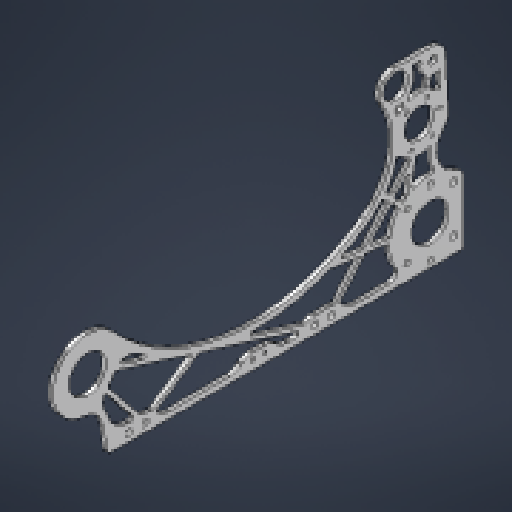
# Autodesk Inventor part: PLATE,SHOOTER,SIDE
Saved by Autodesk Inventor 2026 (Build 300175000, 175)
## iProperties
Created: 2026-01-27
Part Number: PLATE,SHOOTER,SIDE
Material: Aluminum 6061
Document SubType Name: Sheet Metal
Designer: Owen L
Density: 2.7 g/cm^3
Sheet Metal Rule: Default
Appearance: Aluminum - Flat
Mass: 86.5939 g
Surface Area: 289.582 cm^2
Volume: 32.0718 cm^3
Author: Owen L
Autodesk Inventor part; units mm, degrees
ref_plane "YZ Plane" through (0, 0, 0) normal (1, 0, 0) x (0, 1, 0)
ref_plane "XZ Plane" through (0, 0, 0) normal (0, 1, 0) x (-1, 0, 0)
ref_plane "XY Plane" through (0, 0, 0) normal (0, 0, 1) x (1, 0, 0)
sketch "Sketch1" plane through (0, 0, 0) normal (1, 0, 0) x (0, 0, -1)
  circle A0 centre (0, 0) radius 50.8 construction
  arc A1 (166.896579, -77.825153) -> (181.352348, 31.977312) centre (0, 0) ccw construction
  line L0 (0, 0) -> (181.352348, 31.977312) construction
  line L1 (0, 0) -> (184.15, 0) construction
  line L2 (0, 0) -> (166.896579, -77.825153) construction
  arc A2 (207.917963, -26.102167) -> (206.366465, 36.387976) centre (0, 0) ccw construction
  line L3 (0, 0) -> (207.917963, -26.102167) construction
  line L4 (0, 0) -> (206.366465, 36.387976) construction
  circle A3 centre (206.366465, 36.387976) radius 25.4 construction
  circle A4 centre (207.917963, -26.102167) radius 25.4 construction
  arc A5 (206.366465, 36.387976) -> (148.174226, 148.174226) centre (0, 0) ccw construction
  line L5 (0, 0) -> (148.174226, 148.174226) construction
  line L6 (0, 0) -> (206.366465, 36.387976) construction
  arc A6 (185.021668, 98.377766) -> (148.174226, 148.174226) centre (0, 0) ccw construction
  line L7 (0, 0) -> (185.021668, 98.377766) construction
  line L8 (0, 0) -> (148.174226, 148.174226) construction
  circle A7 centre (185.021668, 98.377766) radius 25.4 construction
  circle A8 centre (148.174226, 148.174226) radius 25.4 construction
  circle A9 centre (236.638695, 73.025) radius 15.24 construction
  line L9 (238.323441, -60.809535) -> (238.323441, -0.484535) construction
  line L10 (238.323441, -0.484535) -> (289.123441, -0.484535) construction
  line L11 (289.123441, -0.484535) -> (289.123441, -60.809535) construction
  line L12 (289.123441, -60.809535) -> (238.323441, -60.809535) construction
  line L13 (238.323441, -60.809535) -> (289.123441, -0.484535) construction
  line L14 (238.323441, -0.484535) -> (289.123441, -60.809535) construction
  arc A10 (20.00669, 18.112358) -> (-2.035294, -26.910643) centre (0, 0) ccw
  circle A11 centre (254.497893, 39.37) radius 11 construction
  arc A12 (226.944273, -60.809535) -> (220.780781, 80.357633) centre (0, 0) ccw construction
  line L15 (0, 0) -> (226.944273, -60.809535) construction
  line L16 (0, 0) -> (220.780781, 80.357633) construction
  line L17 (226.944273, -60.809535) -> (16.073441, -60.809535)
  arc A13 (12.401297, -39.983769) -> (-2.035294, -26.910643) centre (-3.232526, -42.740434) ccw
  circle A14 centre (265.213695, 76.2) radius 3.175 construction
  arc A15 (274.718944, 76.813082) -> (265.213695, 85.725) centre (265.213695, 76.2) ccw
  arc A16 (236.638695, 85.725) -> (225.987579, 66.108084) centre (236.638695, 73.025) ccw
  line L18 (265.213695, 85.725) -> (236.638695, 85.725)
  line L19 (271.597527, 53.115395) -> (274.951571, 31.433981) construction
  line L20 (274.951571, 31.433981) -> (257.851938, 17.688586) construction
  line L21 (257.851938, 17.688586) -> (237.39826, 25.624605) construction
  line L22 (237.39826, 25.624605) -> (234.044216, 47.306019) construction
  line L23 (234.044216, 47.306019) -> (251.143849, 61.051414) construction
  line L24 (251.143849, 61.051414) -> (271.597527, 53.115395) construction
  line L25 (273.274549, 42.274688) -> (235.721238, 36.465312) construction
  line L26 (289.123441, -60.809535) -> (226.944273, -60.809535)
  line L27 (16.073441, -60.809535) -> (12.401297, -39.983769)
  line L28 (16.073441, -60.809535) -> (37.220478, -60.809535) construction
  line L29 (244.473589, 51.840498) -> (254.497893, 39.37) construction
  arc A17 (274.653274, 28.323435) -> (283.677721, -5.519175) centre (289.123441, 14.057508) ccw
  arc A18 (274.653274, 28.323435) -> (277.375632, 35.62367) centre (267.870384, 35.010588) ccw
  line L30 (289.123441, -60.809535) -> (289.123441, -12.686522)
  arc A19 (289.123441, -12.686522) -> (283.677721, -5.519175) centre (281.683954, -12.686522) ccw
  arc A20 (212.772408, -2.995184) -> (225.987579, 66.108084) centre (183.383114, 38.440421) ccw
  arc A21 (20.00669, 18.112358) -> (212.772408, -2.995184) centre (128.278186, 116.132181) ccw
  line L31 (236.638695, 73.025) -> (225.987579, 66.108084) construction
  line L32 (274.718944, 76.813082) -> (277.375632, 35.62367)
  point P0 (263.723441, -30.647035)
  point P1 (263.723441, -30.647035)
  point P2 (263.723441, -30.647035)
  point P3 (263.723441, -30.647035)
  point P4 (263.723441, -5.247035)
  point P5 (245.762929, -12.686522)
  point P6 (238.323441, -30.647035)
  point P7 (245.762929, -48.607547)
  point P8 (263.723441, -56.047035)
  point P9 (281.683954, -48.607547)
  point P10 (289.123441, -30.647035)
  point P11 (238.685973, 36.923947)
  point P12 (248.710277, 24.453449)
  point P13 (264.522198, 26.899502)
  point P14 (270.309814, 41.816053)
  point P15 (260.28551, 54.286551)
  dimension "d0" = 101.6
  dimension "d1" = 184.15
  dimension "d2" = 10
  dimension "d3" = 35
  dimension "d4" = 209.55
  dimension "d10" = 35
  dimension "d11" = 17
  dimension "d12" = 50.8
  dimension "d13" = 30.48
  dimension "d14" = 247.65
  dimension "d15" = 50.8
  dimension "d16" = 60.325
  dimension "d17" = 265.4982
  dimension "d19" = 26.9875
  dimension "d20" = 73.025
  dimension "d21" = 22
  dimension "d23" = 38.1
  dimension "d26" = 234.95
  dimension "d27" = 35
  dimension "d28" = 20
  dimension "d30" = 39.37
  dimension "d34" = 6.35
  dimension "d35" = 9.525
  dimension "d36" = 12.7
  dimension "d37" = 76.2
  dimension "d38" = 28.575
  dimension "d39" = 38
  dimension "d40" = 41.275
  dimension "d42" = 273.05
  dimension "d43" = 100
  dimension "d44" = 15.875
  dimension "d45" = 25.4
  dimension "d48" = 360
  dimension "d50" = 16
  dimension "d53" = 360
  dimension "d99" = 62.5094
  dimension "d100" = 20.32
  dimension "d101" = 9.525
  dimension "d102" = 50.8
  dimension "d103" = 33
  dimension "d104" = 146.05
  constraints: 68 end point, 28 point on circle, 22 centre point, 20 coincident, 12 tangent, 6 midpoint, 3 equal radius, 3 horizontal, 3 perpendicular, 2 collinear, 2 equal length, 2 parallel, 2 vertical alignment, 1 line through centre, 1 point on line, 1 vertical, 29 other
  measures "d0" diameter of A0
  measures "d1" radius of A1
  measures "d2" angle of L1 L0
  measures "d3" angle of L2 L0
  measures "d4" radius of A2
  measures "d10" angle of L6 L5
  measures "d11" angle of L7 L8
  measures "d12" diameter of A8
  measures "d13" diameter of A9
  measures "d14" distance of point (0, 0) A9.centre
  measures "d15" distance of L9.end L10.end
  measures "d16" distance of L9.start L9.end
  measures "d17" distance of point (0, 0) point (263.723, -30.647)
  measures "d19" radius of A10
  measures "d20" vertical distance of point (0, 0) A9.centre
  measures "d21" diameter of A11
  measures "d23" distance of A9.centre A11.centre
  measures "d26" radius of A12
  measures "d27" angle of L15 L16
  measures "d28" angle of L1 L16
  measures "d30" distance from line of L1 A11.centre
  measures "d34" diameter of A14
  measures "d35" radius of A15
  measures "d36" radius of A16
  measures "d37" distance from line of A15.centre L1
  measures "d38" horizontal distance of A9.centre A14.centre
  measures "d39" distance between parallel lines of L22 L19
  measures "d40" distance of L32.start L32.end
  measures "d42" distance of L11.end L17.end
  measures "d43" angle of L28 L27
  measures "d44" radius of A13
  measures "d45" distance of point (263.723, -30.647) point (263.723, -5.247)
  measures "d50" distance of L29.start L29.end
  measures "d99" distance of A4.centre L6.end
  measures "d100" radius of A17
  measures "d101" radius of A18
  measures "d102" radius of A20
  measures "d103" angle of L1 L31
  measures "d104" radius of A21
extrude "Plate1" add sketch "Sketch1" along normal blind 3.175
hole "Hole1" at (0, 0, 0) at (0, -30.647035, -263.723441) direction (1, 0, 0) diameter 28.575 end through all
hole "Hole2" at (0, -30.647035, -263.723441) at (0, 73.025, -236.638695) direction (1, 0, 0) diameter 19.05 end through all
hole "Hole3" at (0, 39.37, -254.497893) at (0, -30.647035, -263.723441) direction (1, 0, 0) diameter 22.5 end through all
hole "Hole4" at (0, -12.686522, -281.683954) at (0, -48.607547, -281.683954) at (0, -56.047035, -263.723441) at (0, -48.607547, -245.762929) at (0, -12.686522, -245.762929) at (0, -5.247035, -263.723441) at (0, -30.647035, -263.723441) direction (1, 0, 0) diameter 4.9784 end through all clearance for "Flat Head Machine Screw (82)" size "#10" standard "Ansi Unified Screw Threads"
hole "Hole5" at (0, 51.840498, -244.473589) at (0, 24.453449, -248.710277) at (0, 41.816053, -270.309814) at (0, 54.286551, -260.28551) at (0, 26.899502, -264.522198) direction (1, 0, 0) diameter 3.2004 end through all clearance for "Flat Head Machine Screw" size "M3" standard "Ansi Metric M Profile"
hole "Hole6" at (0, 76.2, -265.213695) direction (1, 0, 0) diameter 6.5278 end through all clearance for "Flat Head Machine Screw (82)" size "1/4" standard "Ansi Unified Screw Threads"
sketch "Sketch2" plane through (3.175, 0, 0) normal (1, 0, 0) x (0, 0, -1)
  line L0 (289.123441, -60.809535) -> (16.073441, -60.809535)
  line L1 (174.823441, -54.459535) -> (187.523441, -54.459535) construction
  line L2 (31.948441, -54.459535) -> (44.648441, -54.459535) construction
  point P0 (0, 0)
  dimension "d106" = 12.7
  dimension "d107" = 6.35
  dimension "d108" = 15.875
  dimension "d110" = 101.6
  constraints: 4 end point, 3 horizontal alignment, 2 horizontal, 1 collinear
  measures "d106" distance of L2.end L2.start
  measures "d107" distance from line of L0 L2.start
  measures "d108" horizontal distance of L0.end L2.start
  measures "d110" horizontal distance of L0.start L1.end
hole "Hole7" at (3.175, -54.459535, -31.948441) at (3.175, -54.459535, -44.648441) at (3.175, -54.459535, -174.823441) at (3.175, -54.459535, -187.523441) direction (-1, 0, 0) diameter 4.9784 depth 3.175 clearance for "Flat Head Machine Screw (82)" size "#10" standard "Ansi Unified Screw Threads"
sketch "Sketch4" plane through (0, 0, 0) normal (-1, 0, 0) x (0, 0, 1)
  line L0 (-16.073441, -60.809535) -> (-289.123441, -60.809535)
  line L1 (-289.123441, -60.809535) -> (-289.123441, -12.686522)
  point P0 (0, 0)
  point P1 (-136.723441, -53.672135)
  point P2 (-127.198441, -53.672135)
  dimension "d144" = 7.1374
  dimension "d145" = 9.525
  dimension "d146" = 152.4
  constraints: 1 horizontal alignment
  measures "d144" distance from line of L0 point (-136.723, -53.672)
  measures "d145" distance of point (-127.198, -53.672) point (-136.723, -53.672)
  measures "d146" distance from line of L1 point (-136.723, -53.672)
hole "Hole8" at (0, -53.672135, -136.723441) at (0, -53.672135, -127.198441) direction (1, 0, 0) diameter 3.242 end through all thread size "M4x0.7" class "6H" standard "ANSI Metric M Profile"
sketch "Sketch3" plane through (0, 0, 0) normal (-1, 0, 0) x (0, 0, 1)
  circle A0 centre (-187.523441, -54.459535) radius 2.4892
  circle A1 centre (-174.823441, -54.459535) radius 2.4892
  circle A2 centre (-44.648441, -54.459535) radius 2.4892
  circle A3 centre (-31.948441, -54.459535) radius 2.4892
  circle A4 centre (-265.213695, 76.2) radius 3.2639
  circle A5 centre (-264.522198, 26.899502) radius 1.6002
  circle A6 centre (-260.28551, 54.286551) radius 1.6002
  circle A7 centre (-270.309814, 41.816053) radius 1.6002
  circle A8 centre (-248.710277, 24.453449) radius 1.6002
  circle A9 centre (-244.473589, 51.840498) radius 1.6002
  circle A10 centre (-263.723441, -5.247035) radius 2.4892
  circle A11 centre (-245.762929, -12.686522) radius 2.4892
  circle A12 centre (-245.762929, -48.607547) radius 2.4892
  circle A13 centre (-263.723441, -56.047035) radius 2.4892
  circle A14 centre (-281.683954, -48.607547) radius 2.4892
  circle A15 centre (-281.683954, -12.686522) radius 2.4892
  circle A16 centre (-254.497893, 39.37) radius 11.25
  circle A17 centre (-236.638695, 73.025) radius 9.525
  circle A18 centre (-263.723441, -30.647035) radius 14.2875
  circle A19 centre (0, 0) radius 14.2875
  arc A20 (-283.677721, -5.519175) -> (-289.123441, -12.686522) centre (-281.683954, -12.686522) ccw
  line L0 (-289.123441, -60.809535) -> (-289.123441, -12.686522)
  line L1 (-16.073441, -60.809535) -> (-289.123441, -60.809535)
  line L2 (-12.401297, -39.983769) -> (-16.073441, -60.809535)
  arc A21 (2.035294, -26.910643) -> (-12.401297, -39.983769) centre (3.232526, -42.740434) ccw
  arc A22 (2.035294, -26.910643) -> (-20.00669, 18.112358) centre (0, 0) ccw
  arc A23 (-212.772408, -2.995184) -> (-20.00669, 18.112358) centre (-128.278186, 116.132181) ccw
  arc A24 (-225.987579, 66.108084) -> (-212.772408, -2.995184) centre (-183.383114, 38.440421) ccw
  arc A25 (-225.987579, 66.108084) -> (-236.638695, 85.725) centre (-236.638695, 73.025) ccw
  line L3 (-265.213695, 85.725) -> (-236.638695, 85.725)
  arc A26 (-265.213695, 85.725) -> (-274.718944, 76.813082) centre (-265.213695, 76.2) ccw
  line L4 (-277.375632, 35.62367) -> (-274.718944, 76.813082)
  arc A27 (-277.375632, 35.62367) -> (-274.653274, 28.323435) centre (-267.870384, 35.010588) ccw
  arc A28 (-283.677721, -5.519175) -> (-274.653274, 28.323435) centre (-289.123441, 14.057508) ccw
  arc A29 (-215.527655, -6.879772) -> (-38.824525, -5.286322) centre (-128.278186, 116.132181) ccw
  arc A30 (1.676125, -22.161706) -> (-16.476097, 14.91606) centre (0, 0) ccw
  arc A31 (-14.095273, -31.530894) -> (-17.091444, -39.15677) centre (3.232526, -42.740434) ccw
  line L5 (-17.091444, -39.15677) -> (-20.069653, -56.047035)
  line L6 (-20.069653, -56.047035) -> (-284.360941, -56.047035)
  line L7 (-284.360941, -56.047035) -> (-284.360941, -12.686522)
  arc A32 (-282.401381, -10.10746) -> (-284.360941, -12.686522) centre (-281.683954, -12.686522) ccw
  arc A33 (-282.401381, -10.10746) -> (-271.261829, 31.667012) centre (-289.123441, 14.057508) ccw
  arc A34 (-272.623008, 35.317129) -> (-271.261829, 31.667012) centre (-267.870384, 35.010588) ccw
  line L8 (-272.623008, 35.317129) -> (-269.966319, 76.506541)
  arc A35 (-265.213695, 80.9625) -> (-269.966319, 76.506541) centre (-265.213695, 76.2) ccw
  line L9 (-265.213695, 80.9625) -> (-236.638695, 80.9625)
  arc A36 (-229.981747, 68.701928) -> (-236.638695, 80.9625) centre (-236.638695, 73.025) ccw
  arc A37 (-229.981747, 68.701928) -> (-215.527655, -6.879772) centre (-183.383114, 38.440421) ccw
  circle A38 centre (-187.523441, -54.459535) radius 6.35
  circle A39 centre (-174.823441, -54.459535) radius 6.35
  circle A40 centre (-44.648441, -54.459535) radius 6.35
  circle A41 centre (-31.948441, -54.459535) radius 6.35
  circle A42 centre (-245.762929, -48.607547) radius 6.35
  circle A43 centre (-245.762929, -12.686522) radius 6.35
  line L10 (-239.412929, -12.686522) -> (-239.412929, -48.607547)
  arc A44 (-239.412929, -48.607547) -> (-231.973441, -56.047035) centre (-231.973441, -48.607547) ccw
  arc A45 (-219.666363, -3.63947) -> (-239.412929, -12.686522) centre (-227.467155, -12.686522) ccw
  line L11 (-187.523441, -48.109535) -> (-174.823441, -48.109535)
  line L12 (-44.648441, -48.109535) -> (-31.948441, -48.109535)
  arc A46 (-31.948441, -48.109535) -> (-16.497451, -36.687798) centre (-31.948441, -31.947843) ccw
  arc A47 (-165.6009, -52.078285) -> (-174.823441, -48.109535) centre (-174.823441, -60.809535) ccw
  arc A48 (-165.6009, -52.078285) -> (-156.378358, -56.047035) centre (-156.378358, -43.347035) ccw
  arc A49 (-44.648441, -48.109535) -> (-53.870983, -52.078285) centre (-44.648441, -60.809535) ccw
  arc A50 (-63.093524, -56.047035) -> (-53.870983, -52.078285) centre (-63.093524, -43.347035) ccw
  arc A51 (-187.523441, -48.109535) -> (-196.745983, -52.078285) centre (-187.523441, -60.809535) ccw
  arc A52 (-205.968524, -56.047035) -> (-196.745983, -52.078285) centre (-205.968524, -43.347035) ccw
  arc A53 (-19.912827, -9.87066) -> (-15.75543, -15.675364) centre (0, 0) ccw
  arc A54 (-19.912827, -9.87066) -> (-38.824525, -5.286322) centre (-31.291586, -15.511038) ccw
  arc A55 (-14.095273, -31.530894) -> (-15.75543, -15.675364) centre (-24.758534, -24.632715) ccw
  line L13 (0, 0) -> (-44.648441, -54.459535) construction
  line L14 (-1.227655, 1.006488) -> (-45.876096, -53.453046)
  line L15 (-43.420786, -55.466023) -> (1.227655, -1.006488)
  arc A56 (1.227655, -1.006488) -> (-1.227655, 1.006488) centre (0, 0) ccw
  arc A57 (-45.876096, -53.453046) -> (-43.420786, -55.466023) centre (-44.648441, -54.459535) ccw
  line L16 (0, 0) -> (-174.823441, -54.459535) construction
  line L17 (-0.472147, 1.515663) -> (-175.295588, -52.943872)
  line L18 (-174.351295, -55.975197) -> (0.472147, -1.515663)
  arc A58 (0.472147, -1.515663) -> (-0.472147, 1.515663) centre (0, 0) ccw
  arc A59 (-175.295588, -52.943872) -> (-174.351295, -55.975197) centre (-174.823441, -54.459535) ccw
  line L19 (-263.723441, -30.647035) -> (0, 0) construction
  line L20 (-263.540193, -32.223923) -> (0.183249, -1.576888)
  line L21 (-0.183249, 1.576888) -> (-263.90669, -29.070147)
  arc A60 (-263.90669, -29.070147) -> (-263.540193, -32.223923) centre (-263.723441, -30.647035) ccw
  arc A61 (0.183249, -1.576888) -> (-0.183249, 1.576888) centre (0, 0) ccw
  line L22 (-44.648441, -54.459535) -> (-236.638695, 73.025) construction
  line L23 (-43.770283, -53.137039) -> (-235.760537, 74.347496)
  line L24 (-237.516853, 71.702504) -> (-45.526599, -55.78203)
  arc A62 (-45.526599, -55.78203) -> (-43.770283, -53.137039) centre (-44.648441, -54.459535) ccw
  arc A63 (-235.760537, 74.347496) -> (-237.516853, 71.702504) centre (-236.638695, 73.025) ccw
  circle A64 centre (-254.497893, 39.37) radius 20.6375
  circle A65 centre (-263.723441, -30.647035) radius 31.75
  line L25 (-254.497893, 39.37) -> (-245.762929, -12.686522) construction
  line L26 (-256.063506, 39.107294) -> (-247.328541, -12.949229)
  line L27 (-244.197317, -12.423816) -> (-252.932281, 39.632706)
  arc A66 (-252.932281, 39.632706) -> (-256.063506, 39.107294) centre (-254.497893, 39.37) ccw
  arc A67 (-247.328541, -12.949229) -> (-244.197317, -12.423816) centre (-245.762929, -12.686522) ccw
  arc A68 (-231.134359, 67.464428) -> (-209.316971, -11.057149) centre (-183.383114, 38.440421) ccw
  circle A69 centre (-270.309814, 41.816053) radius 1.6002
  line L28 (-187.523441, -54.459535) -> (-270.309814, 41.816053) construction
  line L29 (-186.319757, -53.424499) -> (-269.106129, 42.851089)
  line L30 (-271.513498, 40.781017) -> (-188.727126, -55.494571)
  arc A70 (-188.727126, -55.494571) -> (-186.319757, -53.424499) centre (-187.523441, -54.459535) ccw
  arc A71 (-269.106129, 42.851089) -> (-271.513498, 40.781017) centre (-270.309814, 41.816053) ccw
  line L31 (-263.723441, -30.647035) -> (-224.487193, 8.589213) construction
  line L32 (-262.600909, -31.769567) -> (-223.364661, 7.466681)
  line L33 (-225.609725, 9.711745) -> (-264.845973, -29.524503)
  arc A72 (-264.845973, -29.524503) -> (-262.600909, -31.769567) centre (-263.723441, -30.647035) ccw
  arc A73 (-223.364661, 7.466681) -> (-225.609725, 9.711745) centre (-224.487193, 8.589213) ccw
  arc A74 (-225.987579, 66.108084) -> (-212.772408, -2.995184) centre (-183.383114, 38.440421) ccw
  circle A75 centre (-265.213695, 76.2) radius 9.525
  circle A76 centre (-236.638695, 73.025) radius 14.2875
  line L34 (-236.638695, 73.025) -> (-254.497893, 39.37) construction
  line L35 (-238.040986, 73.769133) -> (-255.900185, 40.114133)
  line L36 (-253.095602, 38.625867) -> (-235.236403, 72.280867)
  arc A77 (-235.236403, 72.280867) -> (-238.040986, 73.769133) centre (-236.638695, 73.025) ccw
  arc A78 (-255.900185, 40.114133) -> (-253.095602, 38.625867) centre (-254.497893, 39.37) ccw
  circle A79 centre (-265.213695, 76.2) radius 3.2639
  line L37 (-265.213695, 76.2) -> (-254.497893, 39.37) construction
  line L38 (-266.737987, 75.756503) -> (-256.022185, 38.926503)
  line L39 (-252.973601, 39.813497) -> (-263.689403, 76.643497)
  arc A80 (-263.689403, 76.643497) -> (-266.737987, 75.756503) centre (-265.213695, 76.2) ccw
  arc A81 (-256.022185, 38.926503) -> (-252.973601, 39.813497) centre (-254.497893, 39.37) ccw
  circle A82 centre (-136.723441, -53.672135) radius 4.7625
  circle A83 centre (-127.198441, -53.672135) radius 4.7625
  line L40 (-136.723441, -48.909635) -> (-127.198441, -48.909635)
  arc A84 (-136.723441, -48.909635) -> (-145.550069, -52.478335) centre (-136.723441, -61.609635) ccw
  arc A85 (-154.376697, -56.047035) -> (-145.550069, -52.478335) centre (-154.376697, -43.347035) ccw
  arc A86 (-118.371813, -52.478335) -> (-127.198441, -48.909635) centre (-127.198441, -61.609635) ccw
  arc A87 (-118.371813, -52.478335) -> (-109.545185, -56.047035) centre (-109.545185, -43.347035) ccw
  point P0 (-22.324221, -27.229767)
  point P1 (-87.411721, -27.229767)
  point P2 (-131.861721, -15.323517)
  point P3 (-140.643568, 9.282733)
  point P4 (-13.432223, -18.887743)
  point P5 (-37.389597, -48.109535)
  point P6 (-54.152917, -15.206521)
  point P7 (-23.340411, -5.608067)
  point P8 (-20.921196, -8.179938)
  point P9 (-76.141721, -25.381773)
  point P10 (-82.35281, -27.517637)
  point P11 (-49.738375, -49.174133)
  point P12 (-41.495239, -48.109535)
  point P13 (-15.29981, -16.157896)
  point P14 (-52.720714, -51.005025)
  point P15 (-86.286948, -28.71652)
  point P16 (-90.823459, -29.955305)
  point P17 (-164.676282, -52.961319)
  point P18 (-185.969605, -23.209523)
  point P19 (-167.420127, -50.490574)
  point P20 (-114.70085, -34.067906)
  point P21 (-191.730016, -20.682568)
  point P22 (-239.412929, -26.223751)
  point P23 (-239.412929, -29.420118)
  point P24 (-250.130411, 13.341739)
  point P25 (-237.80423, 27.236246)
  point P26 (-249.527221, 19.340052)
  point P27 (-245.502427, -4.645936)
  point P28 (-239.206177, -10.473631)
  point P29 (-249.086572, -2.472142)
  point P30 (-252.658445, 18.81464)
  point P31 (-265.251466, 21.7556)
  point P32 (-267.806511, 0.839328)
  point P33 (-238.05746, 26.895283)
  point P34 (-228.916628, -6.321741)
  point P35 (-174.823441, -56.047035)
  point P36 (0.472147, -1.515663)
  point P37 (-16.69678, -3.538499)
  point P38 (-40.170203, -6.266322)
  point P39 (-24.96455, -4.499288)
  point P40 (-0.183249, 1.576888)
  point P41 (0.472147, -1.515663)
  point P42 (-252.666593, 18.863196)
  point P43 (-252.62726, 18.817454)
  point P44 (-209.909099, -25.991508)
  point P45 (-190.570963, -48.480601)
  point P46 (-212.407922, -23.085527)
  point P47 (-249.006558, 19.476493)
  point P48 (-216.214904, -23.527932)
  point P49 (-248.666665, 14.211519)
  point P50 (-232.408374, -25.409759)
  point P51 (-193.699263, -49.712273)
  point P52 (-213.716082, -26.433913)
  point P53 (-232.041877, -28.563535)
  point P54 (-239.11127, -50.70454)
  point P55 (-244.105317, -11.028911)
  point P56 (-234.087566, -2.743099)
  point P57 (-238.12774, -7.296397)
  point P58 (-240.17835, -9.347007)
  point P59 (-242.423414, -7.101943)
  point P60 (-235.926268, -0.604798)
  point P61 (-231.598906, -0.767563)
  point P62 (-226.916629, 3.914714)
  point P63 (-233.674843, 1.646628)
  point P64 (-228.836695, 6.484775)
  point P65 (-245.568294, 56.1975)
  point P66 (-259.855794, 57.785)
  point P67 (-241.892133, 59.738389)
  point P68 (-243.450532, 56.801644)
  point P69 (-237.737006, 51.410725)
  point P70 (-235.426451, 58.78902)
  point P71 (-261.770569, 58.683586)
  point P72 (-264.114221, 66.738669)
  point P73 (-270.497264, 68.274754)
  point P74 (-271.618326, 50.893767)
  point P75 (-261.065636, 67.625664)
  point P76 (-258.721985, 59.570581)
  point P77 (-246.255115, 58.289911)
  point P78 (-244.696717, 61.226655)
  point P79 (-248.518457, 80.9625)
  point P80 (-256.964803, 80.9625)
  point P81 (-284.360941, -54.774946)
  point P82 (-282.773441, -56.047035)
  point P83 (-244.673441, -56.047035)
  point P84 (-253.681829, 24.913552)
  point P85 (-249.6819, 20.261876)
  point P86 (-237.492774, 51.06326)
  point P87 (-187.523441, -56.047035)
  point P88 (-187.569806, -51.970766)
  point P89 (-189.977175, -54.040838)
  point P90 (-185.606162, -56.047035)
  point P91 (-189.440721, -56.047035)
  point P92 (-235.071738, 58.823687)
  point P93 (-271.382314, 40.628457)
  point P94 (-268.974945, 42.698529)
  point P95 (-33.865721, -56.047035)
  point P96 (-30.031162, -56.047035)
  point P97 (-176.740721, -56.047035)
  point P98 (-172.906162, -56.047035)
  point P99 (-46.565721, -56.047035)
  point P100 (-42.731162, -56.047035)
  point P101 (-232.948867, 64.243725)
  point P102 (-232.478441, 64.456575)
  point P103 (-230.869647, 67.288655)
  point P104 (-190.328433, -48.762648)
  point P105 (-233.850331, -3.018989)
  dimension "d119" = 12.7
  dimension "d143" = 9.525
  dimension "d118" = 4.7625
  dimension "d120" = 12.7
  dimension "d121" = 12.7
  dimension "d122" = 3.175
  dimension "d123" = 3.175
  dimension "d125" = 3.175
  dimension "d126" = 3.175
  dimension "d130" = 41.275
  dimension "d131" = 63.5
  dimension "d132" = 3.175
  dimension "d133" = 55.88
  dimension "d134" = 3.175
  dimension "d135" = 3.175
  dimension "d136" = 19.05
  dimension "d137" = 28.575
  dimension "d138" = 3.175
  dimension "d139" = 3.175
  dimension "d140" = 9.525
  dimension "d141" = 7.1374
  dimension "d142" = 152.4
  constraints: 95 point on circle, 88 end point, 50 tangent, 48 centre point, 15 equal radius, 14 coincident, 9 midpoint, 9 parallel, 5 vertical alignment, 4 point on line, 3 horizontal, 3 horizontal alignment, 2 vertical, 45 other
  measures "d118" radial gap between concentric circles of A24 A37
  measures "d120" radius of A48
  measures "d121" radius of A54
  measures "d122" diameter of A57
  measures "d123" diameter of A59
  measures "d125" diameter of A61
  measures "d126" diameter of A63
  measures "d130" diameter of A64
  measures "d131" diameter of A65
  measures "d132" diameter of A67
  measures "d133" radius of A68
  measures "d134" diameter of A71
  measures "d135" diameter of A73
  measures "d136" diameter of A75
  measures "d137" diameter of A76
  measures "d138" diameter of A78
  measures "d139" diameter of A81
  measures "d140" distance of point (-127.198, -53.672) point (-136.723, -53.672)
  measures "d141" distance from line of L1 point (-136.723, -53.672)
  measures "d142" distance from line of L0 point (-136.723, -53.672)
sketch "Sketch3 outline for Cut1" plane through (0, 0, 0) normal (-1, 0, 0) x (0, 0, 1)
  arc A0 (-188.727126, -55.494571) -> (-187.523441, -56.047035) centre (-187.523441, -54.459535) ccw
  arc A1 (-187.523441, -56.047035) -> (-186.319757, -53.424499) centre (-187.523441, -54.459535) ccw
  line L0 (-189.977175, -54.040838) -> (-188.727126, -55.494571)
  arc A2 (-187.569806, -51.970766) -> (-189.977175, -54.040838) centre (-187.523441, -54.459535) ccw
  line L1 (-186.319757, -53.424499) -> (-187.569806, -51.970766)
  line L2 (-185.606162, -56.047035) -> (-187.523441, -56.047035)
  line L3 (-187.523441, -56.047035) -> (-189.440721, -56.047035)
  arc A3 (-189.440721, -56.047035) -> (-185.606162, -56.047035) centre (-187.523441, -54.459535) ccw
  line L4 (-261.770569, 58.683586) -> (-264.114221, 66.738669)
  arc A4 (-271.618326, 50.893767) -> (-261.770569, 58.683586) centre (-254.497893, 39.37) cw
  line L5 (-270.497264, 68.274754) -> (-271.618326, 50.893767)
  arc A5 (-264.114221, 66.738669) -> (-270.497264, 68.274754) centre (-265.213695, 76.2) cw
  line L6 (-261.065636, 67.625664) -> (-258.721985, 59.570581)
  arc A6 (-256.964803, 80.9625) -> (-261.065636, 67.625664) centre (-265.213695, 76.2) cw
  line L7 (-248.518457, 80.9625) -> (-256.964803, 80.9625)
  arc A7 (-244.696717, 61.226655) -> (-248.518457, 80.9625) centre (-236.638695, 73.025) cw
  line L8 (-246.255115, 58.289911) -> (-244.696717, 61.226655)
  arc A8 (-258.721985, 59.570581) -> (-246.255115, 58.289911) centre (-254.497893, 39.37) cw
  arc A9 (-235.071738, 58.823687) -> (-241.892133, 59.738389) centre (-236.638695, 73.025) cw
  arc A10 (-237.492774, 51.06326) -> (-235.071738, 58.823687) centre (-183.383114, 38.440421) cw
  arc A11 (-243.450532, 56.801644) -> (-237.492774, 51.06326) centre (-254.497893, 39.37) cw
  line L9 (-241.892133, 59.738389) -> (-243.450532, 56.801644)
  arc A12 (-269.106129, 42.851089) -> (-271.513498, 40.781017) centre (-270.309814, 41.816053) ccw
  line L10 (-268.974945, 42.698529) -> (-269.106129, 42.851089)
  arc A13 (-271.382314, 40.628457) -> (-268.974945, 42.698529) centre (-270.309814, 41.816053) ccw
  line L11 (-271.513498, 40.781017) -> (-271.382314, 40.628457)
  line L12 (-33.865721, -56.047035) -> (-30.031162, -56.047035)
  arc A14 (-30.031162, -56.047035) -> (-33.865721, -56.047035) centre (-31.948441, -54.459535) ccw
  line L13 (-13.432223, -18.887743) -> (-37.389597, -48.109535)
  arc A15 (-14.095273, -31.530894) -> (-13.432223, -18.887743) centre (-24.758534, -24.632715) ccw
  arc A16 (-16.497451, -36.687798) -> (-14.095273, -31.530894) centre (3.232526, -42.740434) cw
  arc A17 (-31.948441, -48.109535) -> (-16.497451, -36.687798) centre (-31.948441, -31.947843) ccw
  line L14 (-37.389597, -48.109535) -> (-31.948441, -48.109535)
  arc A18 (-172.906162, -56.047035) -> (-176.740721, -56.047035) centre (-174.823441, -54.459535) ccw
  line L15 (-176.740721, -56.047035) -> (-172.906162, -56.047035)
  arc A19 (-38.824525, -5.286322) -> (-54.152917, -15.206521) centre (-128.278186, 116.132181) cw
  arc A20 (-23.340411, -5.608067) -> (-38.824525, -5.286322) centre (-31.291586, -15.511038) ccw
  line L16 (-54.152917, -15.206521) -> (-23.340411, -5.608067)
  arc A21 (-42.731162, -56.047035) -> (-46.565721, -56.047035) centre (-44.648441, -54.459535) ccw
  line L17 (-46.565721, -56.047035) -> (-42.731162, -56.047035)
  arc A22 (-231.134359, 67.464428) -> (-232.948867, 64.243725) centre (-183.383114, 38.440421) ccw
  line L18 (-230.869647, 67.288655) -> (-231.134359, 67.464428)
  arc A23 (-232.478441, 64.456575) -> (-230.869647, 67.288655) centre (-183.383114, 38.440421) cw
  arc A24 (-232.948867, 64.243725) -> (-232.478441, 64.456575) centre (-236.638695, 73.025) ccw
  line L19 (-209.909099, -25.991508) -> (-190.328433, -48.762648)
  line L20 (-185.969605, -23.209523) -> (-209.909099, -25.991508)
  arc A25 (-114.70085, -34.067906) -> (-185.969605, -23.209523) centre (-128.278186, 116.132181) cw
  line L21 (-167.420127, -50.490574) -> (-114.70085, -34.067906)
  arc A26 (-174.823441, -48.109535) -> (-167.420127, -50.490574) centre (-174.823441, -60.809535) cw
  line L22 (-187.523441, -48.109535) -> (-174.823441, -48.109535)
  arc A27 (-190.328433, -48.762648) -> (-187.523441, -48.109535) centre (-187.523441, -54.459535) cw
  line L23 (-249.086572, -2.472142) -> (-252.658445, 18.81464)
  arc A28 (-267.806511, 0.839328) -> (-249.086572, -2.472142) centre (-263.723441, -30.647035) cw
  arc A29 (-265.251466, 21.7556) -> (-267.806511, 0.839328) centre (-289.123441, 14.057508) cw
  arc A30 (-252.658445, 18.81464) -> (-265.251466, 21.7556) centre (-254.497893, 39.37) cw
  line L24 (-193.699263, -49.712273) -> (-213.716082, -26.433913)
  arc A31 (-196.745983, -52.078285) -> (-193.699263, -49.712273) centre (-187.523441, -60.809535) cw
  arc A32 (-205.968524, -56.047035) -> (-196.745983, -52.078285) centre (-205.968524, -43.347035) ccw
  line L25 (-231.973441, -56.047035) -> (-205.968524, -56.047035)
  arc A33 (-239.11127, -50.70454) -> (-231.973441, -56.047035) centre (-231.973441, -48.607547) ccw
  arc A34 (-232.041877, -28.563535) -> (-239.11127, -50.70454) centre (-263.723441, -30.647035) cw
  line L26 (-213.716082, -26.433913) -> (-232.041877, -28.563535)
  line L27 (-233.850331, -3.018989) -> (-240.17835, -9.347007)
  line L28 (-216.214904, -23.527932) -> (-233.850331, -3.018989)
  line L29 (-232.408374, -25.409759) -> (-216.214904, -23.527932)
  arc A35 (-240.17835, -9.347007) -> (-232.408374, -25.409759) centre (-263.723441, -30.647035) cw
  line L30 (-226.916629, 3.914714) -> (-231.598906, -0.767563)
  arc A36 (-215.527655, -6.879772) -> (-226.916629, 3.914714) centre (-183.383114, 38.440421) cw
  arc A37 (-191.730016, -20.682568) -> (-215.527655, -6.879772) centre (-128.278186, 116.132181) cw
  line L31 (-212.407922, -23.085527) -> (-191.730016, -20.682568)
  line L32 (-231.598906, -0.767563) -> (-212.407922, -23.085527)
  line L33 (-233.674843, 1.646628) -> (-228.836695, 6.484775)
  line L34 (-249.006558, 19.476493) -> (-233.674843, 1.646628)
  arc A38 (-237.80423, 27.236246) -> (-249.006558, 19.476493) centre (-254.497893, 39.37) cw
  arc A39 (-228.836695, 6.484775) -> (-237.80423, 27.236246) centre (-183.383114, 38.440421) cw
  line L35 (-242.423414, -7.101943) -> (-235.926268, -0.604798)
  arc A40 (-245.502427, -4.645936) -> (-242.423414, -7.101943) centre (-263.723441, -30.647035) cw
  line L36 (-248.666665, 14.211519) -> (-245.502427, -4.645936)
  line L37 (-235.926268, -0.604798) -> (-248.666665, 14.211519)
  arc A41 (-118.371813, -52.478335) -> (-109.545185, -56.047035) centre (-109.545185, -43.347035) ccw
  arc A42 (-127.198441, -48.909635) -> (-118.371813, -52.478335) centre (-127.198441, -61.609635) cw
  line L38 (-136.723441, -48.909635) -> (-127.198441, -48.909635)
  arc A43 (-145.550069, -52.478335) -> (-136.723441, -48.909635) centre (-136.723441, -61.609635) cw
  arc A44 (-154.376697, -56.047035) -> (-145.550069, -52.478335) centre (-154.376697, -43.347035) ccw
  line L39 (-156.378358, -56.047035) -> (-154.376697, -56.047035)
  arc A45 (-164.676282, -52.961319) -> (-156.378358, -56.047035) centre (-156.378358, -43.347035) ccw
  line L40 (-90.823459, -29.955305) -> (-164.676282, -52.961319)
  arc A46 (-86.286948, -28.71652) -> (-90.823459, -29.955305) centre (-128.278186, 116.132181) cw
  line L41 (-52.720714, -51.005025) -> (-86.286948, -28.71652)
  arc A47 (-53.870983, -52.078285) -> (-52.720714, -51.005025) centre (-44.648441, -60.809535) cw
  arc A48 (-63.093524, -56.047035) -> (-53.870983, -52.078285) centre (-63.093524, -43.347035) ccw
  line L42 (-109.545185, -56.047035) -> (-63.093524, -56.047035)
  circle A49 centre (-265.213695, 76.2) radius 3.2639
  arc A50 (-15.75543, -15.675364) -> (-19.912827, -9.87066) centre (0, 0) cw
  arc A51 (-15.29981, -16.157896) -> (-15.75543, -15.675364) centre (-24.758534, -24.632715) ccw
  line L43 (-41.495239, -48.109535) -> (-15.29981, -16.157896)
  line L44 (-44.648441, -48.109535) -> (-41.495239, -48.109535)
  arc A52 (-49.738375, -49.174133) -> (-44.648441, -48.109535) centre (-44.648441, -60.809535) cw
  line L45 (-82.35281, -27.517637) -> (-49.738375, -49.174133)
  arc A53 (-76.141721, -25.381773) -> (-82.35281, -27.517637) centre (-128.278186, 116.132181) cw
  line L46 (-20.921196, -8.179938) -> (-76.141721, -25.381773)
  arc A54 (-19.912827, -9.87066) -> (-20.921196, -8.179938) centre (-31.291586, -15.511038) ccw
extrude "Cut1" cut sketch "Sketch3 outline for Cut1" against normal blind 3.175
fillet "Corner Round1" radius 1.5875 53 edges at (1.5875, -23.2095, -185.9696) (1.5875, -20.6826, -191.73) (1.5875, -50.4906, -167.4201) (1.5875, -52.9613, -164.6763) (1.5875, -60.8095, -16.0734) (1.5875, -34.0679, -114.7008) (1.5875, -29.9553, -90.8235) (1.5875, -28.7165, -86.2869) (1.5875, -25.3818, -76.1417) (1.5875, -27.5176, -82.3528) (1.5875, -51.005, -52.7207) (1.5875, -49.1741, -49.7384) (1.5875, -15.2065, -54.1529) (1.5875, -8.1799, -20.9212) (1.5875, -5.6081, -23.3404) (1.5875, -48.1095, -37.3896) (1.5875, -18.8877, -13.4322) (1.5875, -16.1579, -15.2998) (1.5875, -48.1095, -41.4952) (1.5875, -60.8095, -289.1234) (1.5875, -49.7123, -193.6993) (1.5875, -50.7045, -239.1113) (1.5875, -28.5635, -232.0419) (1.5875, -26.4339, -213.7161) (1.5875, -23.0855, -212.4079) (1.5875, -23.5279, -216.2149) (1.5875, -9.347, -240.1783) (1.5875, 3.9147, -226.9166) (1.5875, -0.7676, -231.5989) (1.5875, 1.6466, -233.6748) (1.5875, 19.4765, -249.0066) (1.5875, 27.2362, -237.8042) (1.5875, 6.4848, -228.8367) (1.5875, 21.7556, -265.2515) (1.5875, 0.8393, -267.8065) (1.5875, -2.4721, -249.0866) (1.5875, 14.2115, -248.6667) (1.5875, -4.6459, -245.5024) (1.5875, -7.1019, -242.4234) (1.5875, -0.6048, -235.9263) (1.5875, 50.8938, -271.6183) (1.5875, 58.6836, -261.7706) (1.5875, 59.5706, -258.722) (1.5875, 68.2748, -270.4973) (1.5875, 66.7387, -264.1142) (1.5875, 67.6257, -261.0656) (1.5875, 80.9625, -256.9648) (1.5875, 80.9625, -248.5185) (1.5875, 61.2267, -244.6967) (1.5875, 58.2899, -246.2551) (1.5875, 56.8016, -243.4505) (1.5875, 59.7384, -241.8921) (1.5875, 18.8146, -252.6584)
equation "\"BendRadius\" = Thickness"
equation "\"BendReliefWidth\" = Thickness"
equation "\"BendReliefDepth\" = 0.5 * Thickness"
equation "\"CornerReliefSize\" = 4 * Thickness"
equation "\"MinimumRemnant\" = 2 * Thickness"
equation "\"TransitionRadius\" = BendRadius"
equation "\"JacobiRadiusSize\" = BendRadius"
equation "\"GapSize\" = Thickness"
equation "\"Thickness\" = 3.175"
body "Solid1"
